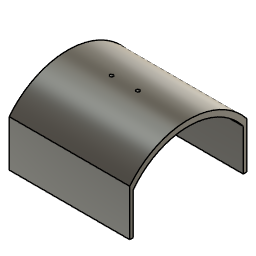
robot top v9 v1 (Autodesk Fusion 360 design; units mm, degrees)
Autodesk Fusion 360 part; units mm, degrees
sketch "Sketch1" plane through (0, 0, 0) normal (1, 0, 0) x (0, 1, 0)
  line L0 (-48, 0) -> (-51, 0)
  line L1 (-48, 0) -> (-51, 0)
  line L2 (48, 0) -> (51, 0)
  line L3 (-51, 0) -> (-51, 40.2989)
  line L4 (51, 0) -> (51, 40.2989)
  arc A0 (48, 36) -> (-48, 36) centre (0, 0) ccw
  arc A1 (51, 40.2989) -> (-51, 40.2989) centre (0, 0) ccw
  line L5 (-51, 0) -> (-48, 0)
  line L6 (-48, 15) -> (-48, 36)
  line L7 (-48, 15) -> (-48, 0)
  line L8 (48, 20.1494) -> (48, 36)
  line L9 (48, 20.1494) -> (48, 0)
  dimension "d1" = 51
  dimension "d2" = 51
  dimension "d3" = 130
  constraint horizontal L0
  constraint parallel L0 L1
  constraint parallel L1 L2
  constraint coincident A0.centre A1.centre
  constraint perpendicular L1 L3
  constraint perpendicular L2 L4
  constraint perpendicular L2 L9
  measures "d1" distance of A0.centre L0.end
  measures "d2" distance of A0.centre L2.end
  measures "d3" diameter of A1
extrude "Extrude1" add sketch "Sketch1" along normal blind 105
hole "Hole1" at (61.1241, 0, 65) direction (0, 0, -1) diameter 3 depth 10 tip angle 118
hole "Hole2" at (38.2805, 0, 65) direction (0, 0, -1) diameter 3 depth 10 tip angle 118
